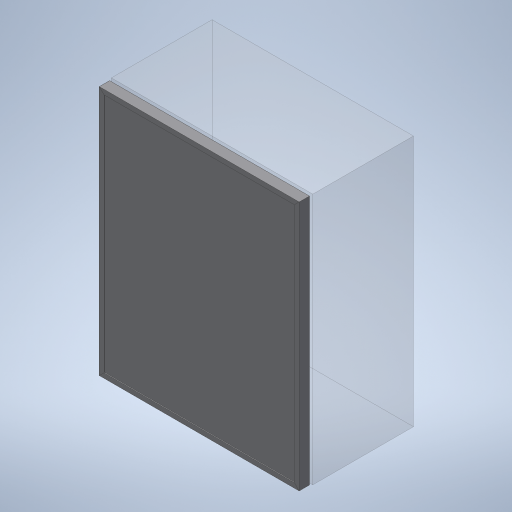
# Autodesk Inventor part: DGL SKELETON
Saved by Autodesk Inventor 2024 (Build 280153000, 153)
## iProperties
RuleStatus: InUse
Created: 2014-05-15
Part Number: DGL SKELETON
Material: Generic
Document SubType Name: Modeling
Designer: SauliusD
Density: 1 g/cm^3
Appearance: Default
Description: Aliuminium Profile Door
Author: SauliusD
Autodesk Inventor part; units mm, degrees
ref_plane "XZ Plane" through (0, 0, 0) normal (0, 1, 0) x (-1, 0, 0)
ref_plane "XY Plane" through (0, 0, 0) normal (0, 0, 1) x (1, 0, 0)
sketch "Sketch11" plane through (0, 0, 0) normal (0, 1, 0) x (-1, 0, 0)
  line L0 (200, -250) -> (-200, -250)
  line L1 (-200, -250) -> (-200, 250)
  line L2 (-200, 250) -> (200, 250)
  line L3 (200, 250) -> (200, -250)
  line L4 (200, -250) -> (-200, 250) construction
  line L5 (-200, -250) -> (200, 250) construction
  point P0 (0, 0)
  dimension "Width" = 400
  dimension "Height" = 500
  constraints: 12 end point, 2 midpoint, 2 parallel, 1 horizontal, 1 perpendicular
  measures "Width" distance of L1.end L2.end
  measures "Height" distance of L0.end L1.end
extrude "Extrusion8" add sketch "Sketch11" along normal blind 200
sketch "Sketch1" plane through (0, 0, 0) normal (0, 1, 0) x (-1, 0, 0)
  line L0 (198.5, -248.5) -> (-198.5, -248.5)
  line L1 (-198.5, -248.5) -> (-198.5, 248.5)
  line L2 (-198.5, 248.5) -> (198.5, 248.5)
  line L3 (198.5, 248.5) -> (198.5, -248.5)
  line L4 (200, 250) -> (200, -250) construction
  line L5 (-200, 250) -> (200, 250) construction
  line L6 (-200, -250) -> (-200, 250) construction
  line L7 (200, -250) -> (-200, -250) construction
  point P0 (0, 0)
  point P1 (0, 248.5)
  point P2 (198.5, 0)
  dimension "Offset_From_Lef" = 1.5
  dimension "Offset_from_Top" = 1.5
  dimension "Offset_from_Bottom" = 1.5
  dimension "Offset_from_Right" = 1.5
  constraints: 8 end point, 2 midpoint, 2 parallel, 1 horizontal, 1 perpendicular
  measures "Offset_From_Lef" distance between parallel lines of L4 L3
  measures "Offset_from_Top" distance between parallel lines of L5 L2
  measures "Offset_from_Bottom" distance between parallel lines of L7 L0
  measures "Offset_from_Right" distance between parallel lines of L6 L1
sketch "Sketch2" plane through (0, 0, 0) normal (0, 1, 0) x (-1, 0, 0)
  line L0 (198.5, 248.5) -> (198.5, -248.5) projected
  line L1 (-198.5, 248.5) -> (198.5, 248.5) projected
  line L2 (-198.5, -248.5) -> (-198.5, 248.5) projected
  line L3 (198.5, -248.5) -> (-198.5, -248.5) projected
  point P0 (0, 0)
ref_plane "Work Plane7" through (198.5, 0, 248.5) normal (1, 0, 0) x (0, 1, 0)
sketch "Sketch3" plane through (198.5, 0, 248.5) normal (1, 0, 0) x (0, 1, 0)
  line L0 (0, 0) -> (-20.5, 0) construction
  line L1 (-20.5, 0) -> (-20.5, -19.05) construction
  line L2 (-20.5, -19.05) -> (0, -19.05) construction
  line L3 (0, -19.05) -> (0, 0) construction
  line L4 (-12.3, 0) -> (0, 0)
  line L5 (0, 0) -> (0, -19.05)
  line L6 (0, -19.05) -> (-12.3, -19.05)
  line L7 (-12.3, -19.05) -> (-12.3, 0)
  line L8 (-12.3, 0) -> (-20.5, 0)
  line L9 (-20.5, 0) -> (-20.5, -1.4)
  line L10 (-20.5, -1.4) -> (-12.3, -1.4)
  line L11 (-12.3, -1.4) -> (-12.3, 0)
  line L12 (-20.5, -1.4) -> (-19.1, -1.4)
  line L13 (-19.1, -1.4) -> (-19.1, -9.4)
  line L14 (-19.1, -9.4) -> (-20.5, -9.4)
  line L15 (-20.5, -9.4) -> (-20.5, -1.4)
  arc A0 (-19.1, -9.4) -> (-19.1, -7.3) centre (-20.437, -8.35) ccw
  arc A1 (-12.3, -16.95) -> (-12.3, -19.05) centre (-10.963, -18) ccw
  point P0 (0, -248.5)
  dimension "Frame_Depth" = 20.5
  dimension "d9" = 19.05
  dimension "d11" = 12.3
  dimension "d13" = 1.4
  dimension "d14" = 1.4
  dimension "d15" = 8
  dimension "d18" = 1.7
  dimension "d19" = 2.1
  dimension "d20" = 2.1
  constraints: 32 end point, 8 parallel, 4 horizontal, 4 perpendicular, 4 point on circle, 4 point on line, 2 centre point, 1 equal radius
  measures "Frame_Depth" distance of L0.start L0.end
  measures "d9" distance of L0.end L1.end
  measures "d11" distance of L2.end L6.end
  measures "d13" distance of L8.end L9.end
  measures "d14" distance of L13.end L14.end
  measures "d15" distance of L12.end L13.end
  measures "d18" radius of A0
  measures "d19" distance from line of L14 A0.end
  measures "d20" distance of A1.start L6.end
sweep "Sweep1" add profiles "Sketch3" path "Sketch1" separate body path curves L2 L3 L0 L1 contours L4 L5 L6 L7
shell "Shell1" thickness 1.4 removed faces 0 bodies 2
sweep "Sweep2" add profiles "Sketch3" path "Sketch2" bodies 2 path curves L1 L0 L3 L2 contours L7 L10 L9 L8 | L7 A1 | L13 L14 L15 L10 | A0 L13
sketch "Sketch6" plane through (-198.5, 0, 248.5) normal (0, 1, 0) x (1, 0, 0)
  line L0 (0, 0) -> (397, 0) projected
  line L1 (397, 497) -> (397, 0) projected
  line L2 (0, 497) -> (397, 497) projected
  line L3 (0, 0) -> (0, 497) projected
  line L4 (19.05, 19.05) -> (19.05, 477.95) projected
  line L5 (19.05, 477.95) -> (377.95, 477.95) projected
  line L6 (377.95, 477.95) -> (377.95, 19.05) projected
  line L7 (377.95, 19.05) -> (19.05, 19.05) projected
  line L8 (377.95, 19.05) -> (397, 0)
  line L9 (19.05, 19.05) -> (0, 0)
  point P0 (198.5, 248.5)
  constraints: 4 end point
extrude "Extrusion2" add sketch "Sketch6" against normal up to surface (20.5 mm away) separate body contours L9 L7 L8 L0
combine bodies "Combine1" operation type common bodies to combine 3 2 keep tools yes
sketch "Sketch7" plane through (-198.5, 0, 248.5) normal (0, 1, 0) x (1, 0, 0)
  line L0 (0, 0) -> (397, 0) projected
  line L1 (397, 497) -> (397, 0) projected
  line L2 (0, 497) -> (397, 497) projected
  line L3 (0, 0) -> (0, 497) projected
  line L4 (19.05, 19.05) -> (19.05, 477.95) projected
  line L5 (19.05, 477.95) -> (377.95, 477.95) projected
  line L6 (377.95, 477.95) -> (377.95, 19.05) projected
  line L7 (377.95, 19.05) -> (19.05, 19.05) projected
  line L8 (377.95, 19.05) -> (397, 0)
  line L9 (397, 497) -> (377.95, 477.95)
  line L10 (387.6, 487.6) -> (388.65, 488.65) projected
  line L11 (0, 0) -> (397, 0) projected
  line L12 (397, 0) -> (377.95, 19.05) projected
  line L13 (377.95, 19.05) -> (19.05, 19.05) projected
  line L14 (19.05, 19.05) -> (0, 0) projected
  point P0 (198.5, 248.5)
  constraints: 4 end point, 1 collinear
extrude "Extrusion3" add sketch "Sketch7" against normal up to surface (20.5 mm away) separate body contours L8 L6 L9 L1
combine bodies "Combine2" operation type common bodies to combine 4 2 keep tools yes
ref_plane "Work Plane10" through (0, 0, 248.5) normal (-1, 0, 0) x (0, -1, 0)
ref_plane "Work Plane11" through (-198.5, 0, 0) normal (0, 0, -1) x (-1, 0, 0)
mirror "Mirror3" about plane through (-198.5, 0, 0) normal (0, 0, -1) bodies 3 separate body
mirror "Mirror4" about plane through (0, 0, 248.5) normal (-1, 0, 0) bodies 4 separate body
sketch "Sketch10" plane through (-197.1, -19.1, 247.1) normal (1, 0, 0) x (0, 0, -1)
  line L0 (0, 0) -> (494.2, 0) projected
  line L1 (494.2, 6.8) -> (494.2, 0) projected
  line L2 (0, 6.8) -> (494.2, 6.8) projected
  line L3 (0, 6.8) -> (0, 0) projected
  point P0 (247.1, 19.1)
extrude "Extrusion7" add sketch "Sketch10" along normal up to surface (394.2 mm away) separate body
move or copy body "Move11" bodies to move or copy 7 3 4 5 6 copy no translate (0, -4.9999, 0)
equation "\"d14\" = d13"
equation "\"d20\" = d19"
equation "\"d95\" = Total_Offset"
equation "\"Total_Offset\" = 4.9999"
equation "\"Inset_Offset\" = 0"
body "Solid1"
